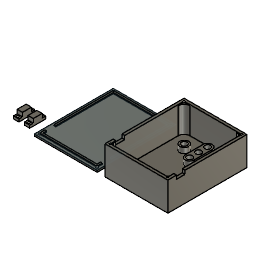
Shutter Tester Laser Enclosure2 (Autodesk Fusion 360 design; units mm, degrees)
Autodesk Fusion 360 part; units mm, degrees
note: some values were not read from the file. Chosen so that the rebuilt part matches the saved one: which bodies a step acts on.
sketch "Sketch1" plane through (0, 0, 0) normal (0, 0, 1) x (1, 0, 0)
  line L0 (-25, -58) -> (45, -58)
  line L1 (45, -58) -> (45, 30)
  line L2 (45, 30) -> (-25, 30)
  line L3 (-25, 30) -> (-25, -58)
  line L4 (-22, 25.9) -> (-22, -53.2245)
  line L5 (-20.782, -55) -> (40.7, -55)
  line L6 (42, -52.82) -> (42, 25.9)
  line L7 (40.7125, 27) -> (-20.7096, 27)
  circle A0 centre (41.997, 27.2) radius 1.3
  circle A1 centre (-21.9941, 27.2) radius 1.3
  line L8 (40, -53) -> (40, 25)
  line L9 (40, 25) -> (-20, 25)
  line L10 (-20, 25) -> (-20, -53)
  line L11 (-20, -53) -> (40, -53)
  line L12 (-22, -53.2245) -> (-22, -53.7)
  line L13 (42, -52.82) -> (42, -53.7)
  circle A2 centre (-22, -55) radius 1.3
  circle A3 centre (42, -55) radius 1.3
  dimension "d23" = 2.6
  dimension "d24" = 2.6
  dimension "d142" = 2.6
  dimension "d143" = 2.6
  constraint horizontal L0
  constraint vertical L1
  constraint horizontal L2
  constraint vertical L3
  constraint coincident A0 L6.end
  constraint coincident A0 L7.start
  constraint coincident A1 L4.start
  constraint coincident A1 L7.end
  constraint parallel L4 L12
  constraint coincident A2 L12.end
  constraint coincident A3 L5.end
  constraint coincident A3 L13.end
  measures "d23" diameter of A0
  measures "d24" diameter of A1
  measures "d142" diameter of A2
  measures "d143" diameter of A3
extrude "Extrude5" add sketch "Sketch1" along normal blind 2 makes body 1 at (-23.732, 0.7336, 2) makes body 2 at (20, -27, 0)
extrude "Extrude6" add sketch "Sketch1" along normal blind 3 contours L4 L5 L6 L7 A0 A1 L12 L13 A2 A3 bodies 1 2
sketch "pcb/cable recess" plane through (0, 0, 3) normal (0, 0, 1) x (-1, 0, 0)
  line L0 (20.7, 55) -> (-40.7, 55)
  line L1 (-42, 53.7) -> (-42, -25.9)
  arc A0 (-40.7125, -27) -> (-42, -25.9) centre (-41.997, -27.2) ccw
  line L2 (-40.7125, -27) -> (20.7096, -27)
  arc A1 (22, -25.9) -> (20.7096, -27) centre (21.9941, -27.2) ccw
  line L3 (22, -25.9) -> (22, 53.2245)
  line L4 (20, 49) -> (22, 49)
  line L5 (22, 49) -> (22, 39)
  line L6 (22, 39) -> (20, 39)
  line L7 (20, 39) -> (20, 49)
  line L8 (-40, 49) -> (-42, 49)
  line L9 (-42, 49) -> (-42, 39)
  line L10 (-42, 39) -> (-40, 39)
  line L11 (-40, 39) -> (-40, 49)
  line L12 (-40, 53) -> (20, 53)
  line L13 (20, 53) -> (20, -25)
  line L14 (20, -25) -> (-40, -25)
  line L15 (-40, -25) -> (-40, 53)
  line L16 (22, 53.2245) -> (22, 53.7)
  arc A2 (-42, 53.7) -> (-40.7, 55) centre (-42, 55) ccw
  arc A3 (20.7, 55) -> (22, 53.7) centre (22, 55) ccw
  constraint horizontal L4
  constraint vertical L5
  constraint horizontal L6
  constraint vertical L7
  constraint horizontal L8
  constraint vertical L9
  constraint horizontal L10
  constraint vertical L11
extrude "Extrude18" cut sketch "pcb/cable recess" against normal blind 1 contours L1 L8 L9 L10 L11 L15 | L3 L4 L5 L6 L7 L13 bodies 1
sketch "clamps" plane through (0, 0, 0) normal (0, 0, 1) x (1, 0, 0)
  line L0 (-35, -35) -> (-35, -53)
  line L1 (-41, -35) -> (-41, -53)
  line L2 (-47, -35) -> (-47, -53)
  line L3 (-53, -35) -> (-53, -53)
  line L4 (-35, -53) -> (-41, -53)
  line L5 (-47, -53) -> (-53, -53)
  line L6 (-35, -49) -> (-41, -49)
  line L7 (-47, -49) -> (-53, -49)
  line L8 (-35, -39) -> (-41, -39)
  line L9 (-47, -39) -> (-53, -39)
  line L10 (-35, -35) -> (-41, -35)
  line L11 (-47, -35) -> (-53, -35)
  circle A0 centre (-50, -37) radius 1.3
  circle A1 centre (-38, -37) radius 1.3
  circle A2 centre (-50, -51) radius 1.3
  circle A3 centre (-38, -51) radius 1.3
  point P0 (-50, -51)
  point P1 (-50, -37)
  point P2 (-38, -37)
  point P3 (-38, -51)
  point P4 (-38, -51)
  dimension "d113" = 2.6
  dimension "d114" = 2.6
  dimension "d115" = 2.6
  dimension "d116" = 2.6
  constraint horizontal L10
  constraint horizontal L8
  constraint horizontal L6
  constraint parallel L4 L6
  constraint perpendicular L0 L4
  constraint coincident L0 L8.start
  constraint coincident L0 L6.start
  constraint collinear L4 L5
  constraint coincident L1 L6.end
  constraint coincident L2 L7.start
  constraint collinear L6 L7
  constraint coincident L1 L8.end
  constraint coincident L2 L9.start
  constraint collinear L8 L9
  constraint collinear L10 L11
  constraint coincident L3 L9.end
  constraint coincident L3 L7.end
  constraint coincident P1 A0.centre
  constraint coincident P2 A1.centre
  constraint coincident P0 A2.centre
  constraint coincident P4 P3
  measures "d113" diameter of A0
  measures "d114" diameter of A1
  measures "d115" diameter of A2
  measures "d116" diameter of A3
extrude "Extrude11" add sketch "clamps" along normal blind 3 separate body contours L0 L1 L8 L10 | L0 L1 L4 L6 | L2 L3 L9 L11 | L2 L3 L5 L7 makes body 3 at (-36.8021, -50.495, 2) makes body 4 at (-37.9676, -35.7004, 2) makes body 5 at (-49.9676, -35.7004, 2) makes body 6 at (-51.2742, -50.7424, 2)
extrude "Extrude12" add sketch "clamps" along normal blind 7.4 contours L0 L1 L6 L8 | L2 L3 L7 L9 bodies 5 3 6 4
sketch "lid" plane through (0, 0, 0) normal (0, 0, 1) x (1, 0, 0)
  line L0 (123.7589, 30) -> (53.7589, 30)
  line L1 (56.7589, 20.4341) -> (56.7589, -47.9212)
  line L2 (120.7589, -47.9212) -> (120.7589, 21.5618)
  line L3 (115.3192, 27.0016) -> (63.3264, 27.0016)
  arc A0 (63.3264, 27.0016) -> (56.7589, 20.4341) centre (63.3264, 20.4341) ccw
  line L4 (56.7589, 20.4341) -> (56.7589, 27.0016)
  line L5 (63.3264, 27.0016) -> (56.7589, 27.0016)
  arc A1 (120.7589, 21.5618) -> (115.3192, 27.0016) centre (115.3192, 21.5618) ccw
  line L6 (115.3192, 27.0016) -> (120.7589, 27.0016)
  line L7 (120.7589, 27.0016) -> (120.7589, 21.5618)
  line L8 (120.7589, -47.9212) -> (120.8187, -55)
  line L9 (56.7589, -55) -> (56.7589, -47.9212)
  circle A2 centre (74, 10) radius 1.2
  circle A3 centre (90, 10) radius 1.2
  circle A4 centre (105.9341, 10.3022) radius 1.2
  circle A5 centre (90, 20) radius 1.2
  circle A6 centre (90, 0) radius 1.2
  circle A7 centre (90, 20) radius 3.2
  circle A8 centre (74, 10) radius 3.2
  circle A9 centre (90, 10) radius 3.2
  circle A10 centre (105.9341, 10.3022) radius 3.2
  circle A11 centre (90, 0) radius 3.2
  circle A12 centre (74, 10) radius 5
  circle A13 centre (105.9341, 10.3022) radius 5
  line L10 (85, 20) -> (85, 0)
  line L11 (95, 20) -> (95, 0)
  arc A14 (85, 0) -> (95, 0) centre (90, 0) ccw
  arc A15 (85, 10.0036) -> (85, 9.9964) centre (90, 10) ccw
  arc A16 (95, 20) -> (85, 20) centre (90, 20) ccw
  line L12 (87, -35) -> (87, -39)
  line L13 (93, -35) -> (93, -39)
  line L14 (87, -49) -> (87, -53)
  line L15 (93, -49) -> (93, -53)
  line L16 (87, -35) -> (93, -35)
  line L17 (87, -39) -> (93, -39)
  line L18 (87, -53) -> (93, -53)
  circle A17 centre (90, -37) radius 1
  circle A18 centre (90, -51) radius 1
  line L19 (87, -49) -> (93, -49)
  line L20 (123.7589, -58) -> (53.7589, -58)
  line L21 (123.7589, 30) -> (123.7589, -58)
  line L22 (53.7589, 30) -> (53.7589, -58)
  line L23 (56.7589, -55) -> (120.8187, -55)
  arc A19 (56.7589, -49) -> (62.7589, -55) centre (62.7589, -49) ccw
  arc A20 (114.7678, -55) -> (120.7676, -48.9493) centre (114.7678, -49) ccw
  line L24 (53.7589, -39) -> (56.7589, -39)
  line L25 (53.7589, -49) -> (56.7589, -49)
  line L26 (120.7635, -48.4594) -> (123.7589, -48.4341)
  line L27 (74, -39) -> (93, -39)
  line L28 (120.7589, -39) -> (123.7589, -39)
  point P0 (90, 10)
  point P1 (90, 10)
  point P2 (90, 20)
  point P3 (90, 0)
  point P4 (74, 10)
  point P5 (105.9341, 10.3022)
  point P6 (90, -37)
  point P7 (90, -51)
  dimension "d118" = 2.4
  dimension "d119" = 2.4
  dimension "d120" = 2.4
  dimension "d121" = 2.4
  dimension "d122" = 2.4
  dimension "d123" = 6.4
  dimension "d124" = 6.4
  dimension "d125" = 6.4
  dimension "d126" = 6.4
  dimension "d127" = 6.4
  dimension "d128" = 10
  dimension "d130" = 10
  dimension "d131" = 10
  dimension "d132" = 10
  dimension "d135" = 2
  dimension "d136" = 2
  dimension "d140" = 6
  dimension "d141" = 6
  constraint horizontal L0
  constraint tangent L1 A0
  constraint tangent L3 A0
  constraint tangent A0 L4
  constraint tangent A0 L5
  constraint tangent L2 A1
  constraint tangent L3 A1
  constraint tangent A1 L6
  constraint tangent A1 L7
  constraint coincident L8.end L23.end
  constraint coincident L9.start L23.start
  constraint coincident P4 A2.centre
  constraint coincident P1 P0
  constraint coincident P5 A4.centre
  constraint coincident P2 A5.centre
  constraint coincident P3 A6.centre
  constraint concentric A3 A9
  constraint concentric A4 A10
  constraint concentric A6 A11
  constraint concentric A11 A14
  constraint concentric A9 A15
  constraint concentric A2 A12
  constraint concentric A4 A13
  constraint concentric A7 A16
  constraint tangent L10 A14
  constraint tangent L11 A14
  constraint coincident L10 A15.start
  constraint coincident L10 A15.end
  constraint horizontal L17
  constraint perpendicular L15 L18
  constraint coincident P6 A17.centre
  constraint coincident P7 A18.centre
  constraint horizontal L20
  constraint perpendicular L20 L21
  constraint perpendicular L20 L22
  constraint perpendicular L21 L23
  constraint tangent L8 A20
  constraint tangent L23 A20
  constraint tangent L23 A19
  constraint tangent L9 A19
  constraint coincident L23 A19.end
  constraint coincident L9 A19.start
  constraint coincident L8 A20.end
  constraint coincident L23 A20.start
  constraint coincident L1 L24.end
  constraint perpendicular L1 L24
  constraint coincident L21 L28.end
  constraint perpendicular L21 L27
  constraint coincident L21 L26.end
  constraint perpendicular L8 L26
  constraint coincident L22 L24.start
  constraint coincident L22 L25.start
  constraint collinear L27 L28
  constraint coincident L2 L28.start
  constraint coincident L8 L26.start
  measures "d118" diameter of A2
  measures "d119" diameter of A3
  measures "d120" diameter of A4
  measures "d121" diameter of A5
  measures "d122" diameter of A6
  measures "d123" diameter of A7
  measures "d124" diameter of A8
  measures "d125" diameter of A9
  measures "d126" diameter of A10
  measures "d127" diameter of A11
  measures "d128" diameter of A14
  measures "d130" diameter of A12
  measures "d131" diameter of A13
  measures "d132" diameter of A16
  measures "d135" diameter of A17
  measures "d136" diameter of A18
  measures "d140" radius of A20
  measures "d141" radius of A19
extrude "Extrude22" add sketch "lid" along normal blind 2 separate body contours L1 L2 L3 A0 A1 L8 L9 L23 A19 A20 | A7 | A8 | A9 | A10 | A11 | A17 | A18 makes body 7 at (71.9774, -26.2181, 0) makes body 8 at (93.196, -0.1595, 1.3333) makes body 9 at (93.196, 9.8405, 1.3333) makes body 10 at (109.1301, 10.1427, 1.3333) makes body 11 at (77.196, 9.8405, 1.3333) makes body 12 at (93.196, 19.8405, 1.3333) makes body 13 at (90.9215, -36.6116, 1.3333) makes body 14 at (90.766, -50.3572, 1.3333)
extrude "Extrude23" add sketch "lid" along normal blind 8 contours A12 | A13 | L10 L11 A14 A15 A16 | L12 L13 L16 L17 L27 | L14 L15 L18 L19 bodies 7 12 11 10 13 9 8 14
extrude "Extrude24" add sketch "lid" along normal blind 32 contours L0 L1 L2 L3 L4 L5 L6 L7 L21 L22 L24 L28 | L8 L9 L20 L21 L22 L23 L25 L26 bodies 7
extrude "Extrude26" add sketch "lid" along normal blind 28 contours L2 L8 L21 L26 L28 | L1 L9 L22 L24 L25 bodies 7
extrude "Extrude25" add sketch "lid" along normal blind 31 contours A1 L6 L7 | L9 L23 A19 | A0 L4 L5 | L8 L23 A20 bodies 7
hole "Hole7" at (56.7589, 27.0016, 32) at (120.7589, 27.0016, 32) at (120.8187, -55, 32) at (56.7589, -55, 32) direction (0, 0, -1) diameter 2 depth 8 tip angle 180 bodies 7
sketch "Sketch7" plane through (0, 0, 2) normal (0, 0, 1) x (-1, 0, 0)
  line L0 (22, 39) -> (22, -25.9)
  arc A0 (20.7096, -27) -> (22, -25.9) centre (21.9941, -27.2) ccw
  line L1 (20.7096, -27) -> (-40.7125, -27)
  arc A1 (-42, -25.9) -> (-40.7125, -27) centre (-41.997, -27.2) ccw
  line L2 (-42, -25.9) -> (-42, 39)
  line L3 (-42, 39) -> (-40, 39)
  line L4 (-40, 39) -> (-40, -25)
  line L5 (-40, -25) -> (20, -25)
  line L6 (20, -25) -> (20, 39)
  line L7 (20, 39) -> (22, 39)
  line L8 (25, -30) -> (25, 58)
  line L9 (25, 58) -> (-45, 58)
  line L10 (-45, 58) -> (-45, -30)
  line L11 (-45, -30) -> (25, -30)
  line L12 (22, 49) -> (20, 49)
  line L13 (20, 49) -> (20, 53)
  line L14 (20, 53) -> (-40, 53)
  line L15 (-40, 53) -> (-40, 49)
  line L16 (-40, 49) -> (-42, 49)
  line L17 (-42, 49) -> (-42, 53.7)
  arc A2 (-40.7, 55) -> (-42, 53.7) centre (-42, 55) ccw
  line L18 (-40.7, 55) -> (20.7, 55)
  arc A3 (22, 53.7) -> (20.7, 55) centre (22, 55) ccw
  line L19 (22, 53.7) -> (22, 53.2245)
  line L20 (22, 53.2245) -> (22, 49)
named bodies: "clamp1", "clamp2"
